Autodesk Fusion 360 part; units mm, degrees
(part 7 of 12)
  line L1818 (4.0736, 136.7487) -> (8.4037, 134.2487)
  line L1819 (8.4037, 134.2487) -> (12.7339, 136.7487)
  line L1820 (12.7339, 136.7487) -> (12.7339, 141.7487)
  line L1821 (12.7339, 141.7487) -> (8.4037, 144.2487)
  line L1822 (19.064, 144.2487) -> (14.7339, 141.7487)
  line L1823 (14.7339, 141.7487) -> (14.7339, 136.7487)
  line L1824 (14.7339, 136.7487) -> (19.064, 134.2487)
  line L1825 (19.064, 134.2487) -> (23.3941, 136.7487)
  line L1826 (23.3941, 136.7487) -> (23.3941, 141.7487)
  line L1827 (23.3941, 141.7487) -> (19.064, 144.2487)
  line L1828 (29.7242, 144.2487) -> (25.3941, 141.7487)
  line L1829 (25.3941, 141.7487) -> (25.3941, 136.7487)
  line L1830 (25.3941, 136.7487) -> (29.7242, 134.2487)
  line L1831 (29.7242, 134.2487) -> (34.0544, 136.7487)
  line L1832 (34.0544, 136.7487) -> (34.0544, 141.7487)
  line L1833 (34.0544, 141.7487) -> (29.7242, 144.2487)
  line L1834 (40.3845, 144.2487) -> (36.0544, 141.7487)
  line L1835 (36.0544, 141.7487) -> (36.0544, 136.7487)
  line L1836 (36.0544, 136.7487) -> (40.3845, 134.2487)
  line L1837 (40.3845, 134.2487) -> (44.7146, 136.7487)
  line L1838 (44.7146, 136.7487) -> (44.7146, 141.7487)
  line L1839 (44.7146, 141.7487) -> (40.3845, 144.2487)
  line L1840 (51.0447, 144.2487) -> (46.7146, 141.7487)
  line L1841 (46.7146, 141.7487) -> (46.7146, 136.7487)
  line L1842 (46.7146, 136.7487) -> (51.0447, 134.2487)
  line L1843 (51.0447, 134.2487) -> (55.3749, 136.7487)
  line L1844 (55.3749, 136.7487) -> (55.3749, 141.7487)
  line L1845 (55.3749, 141.7487) -> (51.0447, 144.2487)
  line L1846 (61.705, 144.2487) -> (57.3749, 141.7487)
  line L1847 (57.3749, 141.7487) -> (57.3749, 136.7487)
  line L1848 (57.3749, 136.7487) -> (61.705, 134.2487)
  line L1849 (61.705, 134.2487) -> (66.0351, 136.7487)
  line L1850 (66.0351, 136.7487) -> (66.0351, 141.7487)
  line L1851 (66.0351, 141.7487) -> (61.705, 144.2487)
  line L1852 (-146.17, 153.4808) -> (-150.5001, 150.9808)
  line L1853 (-150.5001, 150.9808) -> (-150.5001, 145.9808)
  line L1854 (-150.5001, 145.9808) -> (-146.17, 143.4808)
  line L1855 (-146.17, 143.4808) -> (-141.8398, 145.9808)
  line L1856 (-141.8398, 145.9808) -> (-141.8398, 150.9808)
  line L1857 (-141.8398, 150.9808) -> (-146.17, 153.4808)
  line L1858 (-135.5097, 153.4808) -> (-139.8398, 150.9808)
  line L1859 (-139.8398, 150.9808) -> (-139.8398, 145.9808)
  line L1860 (-139.8398, 145.9808) -> (-135.5097, 143.4808)
  line L1861 (-135.5097, 143.4808) -> (-131.1796, 145.9808)
  line L1862 (-131.1796, 145.9808) -> (-131.1796, 150.9808)
  line L1863 (-131.1796, 150.9808) -> (-135.5097, 153.4808)
  line L1864 (-124.8494, 153.4808) -> (-129.1796, 150.9808)
  line L1865 (-129.1796, 150.9808) -> (-129.1796, 145.9808)
  line L1866 (-129.1796, 145.9808) -> (-124.8494, 143.4808)
  line L1867 (-124.8494, 143.4808) -> (-120.5193, 145.9808)
  line L1868 (-120.5193, 145.9808) -> (-120.5193, 150.9808)
  line L1869 (-120.5193, 150.9808) -> (-124.8494, 153.4808)
  line L1870 (-114.1892, 153.4808) -> (-118.5193, 150.9808)
  line L1871 (-118.5193, 150.9808) -> (-118.5193, 145.9808)
  line L1872 (-118.5193, 145.9808) -> (-114.1892, 143.4808)
  line L1873 (-114.1892, 143.4808) -> (-109.8591, 145.9808)
  line L1874 (-109.8591, 145.9808) -> (-109.8591, 150.9808)
  line L1875 (-109.8591, 150.9808) -> (-114.1892, 153.4808)
  line L1876 (-103.5289, 153.4808) -> (-107.8591, 150.9808)
  line L1877 (-107.8591, 150.9808) -> (-107.8591, 145.9808)
  line L1878 (-107.8591, 145.9808) -> (-103.5289, 143.4808)
  line L1879 (-103.5289, 143.4808) -> (-99.1988, 145.9808)
  line L1880 (-99.1988, 145.9808) -> (-99.1988, 150.9808)
  line L1881 (-99.1988, 150.9808) -> (-103.5289, 153.4808)
  line L1882 (-92.8687, 153.4808) -> (-97.1988, 150.9808)
  line L1883 (-97.1988, 150.9808) -> (-97.1988, 145.9808)
  line L1884 (-97.1988, 145.9808) -> (-92.8687, 143.4808)
  line L1885 (-92.8687, 143.4808) -> (-88.5386, 145.9808)
  line L1886 (-88.5386, 145.9808) -> (-88.5386, 150.9808)
  line L1887 (-88.5386, 150.9808) -> (-92.8687, 153.4808)
  line L1888 (-82.2084, 153.4808) -> (-86.5386, 150.9808)
  line L1889 (-86.5386, 150.9808) -> (-86.5386, 145.9808)
  line L1890 (-86.5386, 145.9808) -> (-82.2084, 143.4808)
  line L1891 (-82.2084, 143.4808) -> (-77.8783, 145.9808)
  line L1892 (-77.8783, 145.9808) -> (-77.8783, 150.9808)
  line L1893 (-77.8783, 150.9808) -> (-82.2084, 153.4808)
  line L1894 (-71.5482, 153.4808) -> (-75.8783, 150.9808)
  line L1895 (-75.8783, 150.9808) -> (-75.8783, 145.9808)
  line L1896 (-75.8783, 145.9808) -> (-71.5482, 143.4808)
  line L1897 (-71.5482, 143.4808) -> (-67.218, 145.9808)
  line L1898 (-67.218, 145.9808) -> (-67.218, 150.9808)
  line L1899 (-67.218, 150.9808) -> (-71.5482, 153.4808)
  line L1900 (-60.8879, 153.4808) -> (-65.218, 150.9808)
  line L1901 (-65.218, 150.9808) -> (-65.218, 145.9808)
  line L1902 (-65.218, 145.9808) -> (-60.8879, 143.4808)
  line L1903 (-60.8879, 143.4808) -> (-56.5578, 145.9808)
  line L1904 (-56.5578, 145.9808) -> (-56.5578, 150.9808)
  line L1905 (-56.5578, 150.9808) -> (-60.8879, 153.4808)
  line L1906 (-50.2277, 153.4808) -> (-54.5578, 150.9808)
  line L1907 (-54.5578, 150.9808) -> (-54.5578, 145.9808)
  line L1908 (-54.5578, 145.9808) -> (-50.2277, 143.4808)
  line L1909 (-50.2277, 143.4808) -> (-45.8975, 145.9808)
  line L1910 (-45.8975, 145.9808) -> (-45.8975, 150.9808)
  line L1911 (-45.8975, 150.9808) -> (-50.2277, 153.4808)
  line L1912 (-39.5674, 153.4808) -> (-43.8975, 150.9808)
  line L1913 (-43.8975, 150.9808) -> (-43.8975, 145.9808)
  line L1914 (-43.8975, 145.9808) -> (-39.5674, 143.4808)
  line L1915 (-39.5674, 143.4808) -> (-35.2373, 145.9808)
  line L1916 (-35.2373, 145.9808) -> (-35.2373, 150.9808)
  line L1917 (-35.2373, 150.9808) -> (-39.5674, 153.4808)
  line L1918 (-28.9072, 153.4808) -> (-33.2373, 150.9808)
  line L1919 (-33.2373, 150.9808) -> (-33.2373, 145.9808)
  line L1920 (-33.2373, 145.9808) -> (-28.9072, 143.4808)
  line L1921 (-28.9072, 143.4808) -> (-24.577, 145.9808)
  line L1922 (-24.577, 145.9808) -> (-24.577, 150.9808)
  line L1923 (-24.577, 150.9808) -> (-28.9072, 153.4808)
  line L1924 (-18.2469, 153.4808) -> (-22.577, 150.9808)
  line L1925 (-22.577, 150.9808) -> (-22.577, 145.9808)
  line L1926 (-22.577, 145.9808) -> (-18.2469, 143.4808)
  line L1927 (-18.2469, 143.4808) -> (-13.9168, 145.9808)
  line L1928 (-13.9168, 145.9808) -> (-13.9168, 150.9808)
  line L1929 (-13.9168, 150.9808) -> (-18.2469, 153.4808)
  line L1930 (-7.5866, 153.4808) -> (-11.9168, 150.9808)
  line L1931 (-11.9168, 150.9808) -> (-11.9168, 145.9808)
  line L1932 (-11.9168, 145.9808) -> (-7.5866, 143.4808)
  line L1933 (-7.5866, 143.4808) -> (-3.2565, 145.9808)
  line L1934 (-3.2565, 145.9808) -> (-3.2565, 150.9808)
  line L1935 (-3.2565, 150.9808) -> (-7.5866, 153.4808)
  line L1936 (3.0736, 153.4808) -> (-1.2565, 150.9808)
  line L1937 (-1.2565, 150.9808) -> (-1.2565, 145.9808)
  line L1938 (-1.2565, 145.9808) -> (3.0736, 143.4808)
  line L1939 (3.0736, 143.4808) -> (7.4037, 145.9808)
  line L1940 (7.4037, 145.9808) -> (7.4037, 150.9808)
  line L1941 (7.4037, 150.9808) -> (3.0736, 153.4808)
  line L1942 (13.7339, 153.4808) -> (9.4037, 150.9808)
  line L1943 (9.4037, 150.9808) -> (9.4037, 145.9808)
  line L1944 (9.4037, 145.9808) -> (13.7339, 143.4808)
  line L1945 (13.7339, 143.4808) -> (18.064, 145.9808)
  line L1946 (18.064, 145.9808) -> (18.064, 150.9808)
  line L1947 (18.064, 150.9808) -> (13.7339, 153.4808)
  line L1948 (24.3941, 153.4808) -> (20.064, 150.9808)
  line L1949 (20.064, 150.9808) -> (20.064, 145.9808)
  line L1950 (20.064, 145.9808) -> (24.3941, 143.4808)
  line L1951 (24.3941, 143.4808) -> (28.7242, 145.9808)
  line L1952 (28.7242, 145.9808) -> (28.7242, 150.9808)
  line L1953 (28.7242, 150.9808) -> (24.3941, 153.4808)
  line L1954 (35.0544, 153.4808) -> (30.7242, 150.9808)
  line L1955 (30.7242, 150.9808) -> (30.7242, 145.9808)
  line L1956 (30.7242, 145.9808) -> (35.0544, 143.4808)
  line L1957 (35.0544, 143.4808) -> (39.3845, 145.9808)
  line L1958 (39.3845, 145.9808) -> (39.3845, 150.9808)
  line L1959 (39.3845, 150.9808) -> (35.0544, 153.4808)
  line L1960 (45.7146, 153.4808) -> (41.3845, 150.9808)
  line L1961 (41.3845, 150.9808) -> (41.3845, 145.9808)
  line L1962 (41.3845, 145.9808) -> (45.7146, 143.4808)
  line L1963 (45.7146, 143.4808) -> (50.0447, 145.9808)
  line L1964 (50.0447, 145.9808) -> (50.0447, 150.9808)
  line L1965 (50.0447, 150.9808) -> (45.7146, 153.4808)
  line L1966 (56.3749, 153.4808) -> (52.0447, 150.9808)
  line L1967 (52.0447, 150.9808) -> (52.0447, 145.9808)
  line L1968 (52.0447, 145.9808) -> (56.3749, 143.4808)
  line L1969 (56.3749, 143.4808) -> (60.705, 145.9808)
  line L1970 (60.705, 145.9808) -> (60.705, 150.9808)
  line L1971 (60.705, 150.9808) -> (56.3749, 153.4808)
  line L1972 (-151.5001, 162.7128) -> (-155.8302, 160.2128)
  line L1973 (-155.8302, 160.2128) -> (-155.8302, 155.2128)
  line L1974 (-155.8302, 155.2128) -> (-151.5001, 152.7128)
  line L1975 (-151.5001, 152.7128) -> (-147.17, 155.2128)
  line L1976 (-147.17, 155.2128) -> (-147.17, 160.2128)
  line L1977 (-147.17, 160.2128) -> (-151.5001, 162.7128)
  line L1978 (-140.8398, 162.7128) -> (-145.17, 160.2128)
  line L1979 (-145.17, 160.2128) -> (-145.17, 155.2128)
  line L1980 (-145.17, 155.2128) -> (-140.8398, 152.7128)
  line L1981 (-140.8398, 152.7128) -> (-136.5097, 155.2128)
  line L1982 (-136.5097, 155.2128) -> (-136.5097, 160.2128)
  line L1983 (-136.5097, 160.2128) -> (-140.8398, 162.7128)
  line L1984 (-130.1796, 162.7128) -> (-134.5097, 160.2128)
  line L1985 (-134.5097, 160.2128) -> (-134.5097, 155.2128)
  line L1986 (-134.5097, 155.2128) -> (-130.1796, 152.7128)
  line L1987 (-130.1796, 152.7128) -> (-125.8494, 155.2128)
  line L1988 (-125.8494, 155.2128) -> (-125.8494, 160.2128)
  line L1989 (-125.8494, 160.2128) -> (-130.1796, 162.7128)
  line L1990 (-119.5193, 162.7128) -> (-123.8494, 160.2128)
  line L1991 (-123.8494, 160.2128) -> (-123.8494, 155.2128)
  line L1992 (-123.8494, 155.2128) -> (-119.5193, 152.7128)
  line L1993 (-119.5193, 152.7128) -> (-115.1892, 155.2128)
  line L1994 (-115.1892, 155.2128) -> (-115.1892, 160.2128)
  line L1995 (-115.1892, 160.2128) -> (-119.5193, 162.7128)
  line L1996 (-108.8591, 162.7128) -> (-113.1892, 160.2128)
  line L1997 (-113.1892, 160.2128) -> (-113.1892, 155.2128)
  line L1998 (-113.1892, 155.2128) -> (-108.8591, 152.7128)
  line L1999 (-108.8591, 152.7128) -> (-104.5289, 155.2128)
  line L2000 (-104.5289, 155.2128) -> (-104.5289, 160.2128)
  line L2001 (-104.5289, 160.2128) -> (-108.8591, 162.7128)
  line L2002 (-98.1988, 162.7128) -> (-102.5289, 160.2128)
  line L2003 (-102.5289, 160.2128) -> (-102.5289, 155.2128)
  line L2004 (-102.5289, 155.2128) -> (-98.1988, 152.7128)
  line L2005 (-98.1988, 152.7128) -> (-93.8687, 155.2128)
  line L2006 (-93.8687, 155.2128) -> (-93.8687, 160.2128)
  line L2007 (-93.8687, 160.2128) -> (-98.1988, 162.7128)
  line L2008 (-87.5386, 162.7128) -> (-91.8687, 160.2128)
  line L2009 (-91.8687, 160.2128) -> (-91.8687, 155.2128)
  line L2010 (-91.8687, 155.2128) -> (-87.5386, 152.7128)
  line L2011 (-87.5386, 152.7128) -> (-83.2084, 155.2128)
  line L2012 (-83.2084, 155.2128) -> (-83.2084, 160.2128)
  line L2013 (-83.2084, 160.2128) -> (-87.5386, 162.7128)
  line L2014 (-76.8783, 162.7128) -> (-81.2084, 160.2128)
  line L2015 (-81.2084, 160.2128) -> (-81.2084, 155.2128)
  line L2016 (-81.2084, 155.2128) -> (-76.8783, 152.7128)
  line L2017 (-76.8783, 152.7128) -> (-72.5482, 155.2128)
  line L2018 (-72.5482, 155.2128) -> (-72.5482, 160.2128)
  line L2019 (-72.5482, 160.2128) -> (-76.8783, 162.7128)
  line L2020 (-66.218, 162.7128) -> (-70.5482, 160.2128)
  line L2021 (-70.5482, 160.2128) -> (-70.5482, 155.2128)
  line L2022 (-70.5482, 155.2128) -> (-66.218, 152.7128)
  line L2023 (-66.218, 152.7128) -> (-61.8879, 155.2128)
  line L2024 (-61.8879, 155.2128) -> (-61.8879, 160.2128)
  line L2025 (-61.8879, 160.2128) -> (-66.218, 162.7128)
  line L2026 (-55.5578, 162.7128) -> (-59.8879, 160.2128)
  line L2027 (-59.8879, 160.2128) -> (-59.8879, 155.2128)
  line L2028 (-59.8879, 155.2128) -> (-55.5578, 152.7128)
  line L2029 (-55.5578, 152.7128) -> (-51.2277, 155.2128)
  line L2030 (-51.2277, 155.2128) -> (-51.2277, 160.2128)
  line L2031 (-51.2277, 160.2128) -> (-55.5578, 162.7128)
  line L2032 (-44.8975, 162.7128) -> (-49.2277, 160.2128)
  line L2033 (-49.2277, 160.2128) -> (-49.2277, 155.2128)
  line L2034 (-49.2277, 155.2128) -> (-44.8975, 152.7128)
  line L2035 (-44.8975, 152.7128) -> (-40.5674, 155.2128)
  line L2036 (-40.5674, 155.2128) -> (-40.5674, 160.2128)
  line L2037 (-40.5674, 160.2128) -> (-44.8975, 162.7128)
  line L2038 (-34.2373, 162.7128) -> (-38.5674, 160.2128)
  line L2039 (-38.5674, 160.2128) -> (-38.5674, 155.2128)
  line L2040 (-38.5674, 155.2128) -> (-34.2373, 152.7128)
  line L2041 (-34.2373, 152.7128) -> (-29.9072, 155.2128)
  line L2042 (-29.9072, 155.2128) -> (-29.9072, 160.2128)
  line L2043 (-29.9072, 160.2128) -> (-34.2373, 162.7128)
  line L2044 (-23.577, 162.7128) -> (-27.9072, 160.2128)
  line L2045 (-27.9072, 160.2128) -> (-27.9072, 155.2128)
  line L2046 (-27.9072, 155.2128) -> (-23.577, 152.7128)
  line L2047 (-23.577, 152.7128) -> (-19.2469, 155.2128)
  line L2048 (-19.2469, 155.2128) -> (-19.2469, 160.2128)
  line L2049 (-19.2469, 160.2128) -> (-23.577, 162.7128)
  line L2050 (-12.9168, 162.7128) -> (-17.2469, 160.2128)
  line L2051 (-17.2469, 160.2128) -> (-17.2469, 155.2128)
  line L2052 (-17.2469, 155.2128) -> (-12.9168, 152.7128)
  line L2053 (-12.9168, 152.7128) -> (-8.5866, 155.2128)
  line L2054 (-8.5866, 155.2128) -> (-8.5866, 160.2128)
  line L2055 (-8.5866, 160.2128) -> (-12.9168, 162.7128)
  line L2056 (-2.2565, 162.7128) -> (-6.5866, 160.2128)
  line L2057 (-6.5866, 160.2128) -> (-6.5866, 155.2128)
  line L2058 (-6.5866, 155.2128) -> (-2.2565, 152.7128)
  line L2059 (-2.2565, 152.7128) -> (2.0736, 155.2128)
  line L2060 (2.0736, 155.2128) -> (2.0736, 160.2128)
  line L2061 (2.0736, 160.2128) -> (-2.2565, 162.7128)
  line L2062 (8.4037, 162.7128) -> (4.0736, 160.2128)
  line L2063 (4.0736, 160.2128) -> (4.0736, 155.2128)
  line L2064 (4.0736, 155.2128) -> (8.4037, 152.7128)
  line L2065 (8.4037, 152.7128) -> (12.7339, 155.2128)
  line L2066 (12.7339, 155.2128) -> (12.7339, 160.2128)
  line L2067 (12.7339, 160.2128) -> (8.4037, 162.7128)
  line L2068 (19.064, 162.7128) -> (14.7339, 160.2128)
  line L2069 (14.7339, 160.2128) -> (14.7339, 155.2128)
  line L2070 (14.7339, 155.2128) -> (19.064, 152.7128)
  line L2071 (19.064, 152.7128) -> (23.3941, 155.2128)
  line L2072 (23.3941, 155.2128) -> (23.3941, 160.2128)
  line L2073 (23.3941, 160.2128) -> (19.064, 162.7128)
  line L2074 (29.7242, 162.7128) -> (25.3941, 160.2128)
  line L2075 (25.3941, 160.2128) -> (25.3941, 155.2128)
  line L2076 (25.3941, 155.2128) -> (29.7242, 152.7128)
  line L2077 (29.7242, 152.7128) -> (34.0544, 155.2128)
  line L2078 (34.0544, 155.2128) -> (34.0544, 160.2128)
  line L2079 (34.0544, 160.2128) -> (29.7242, 162.7128)
  line L2080 (40.3845, 162.7128) -> (36.0544, 160.2128)
  line L2081 (36.0544, 160.2128) -> (36.0544, 155.2128)
  line L2082 (36.0544, 155.2128) -> (40.3845, 152.7128)
  line L2083 (40.3845, 152.7128) -> (44.7146, 155.2128)
  line L2084 (44.7146, 155.2128) -> (44.7146, 160.2128)
  line L2085 (44.7146, 160.2128) -> (40.3845, 162.7128)
  line L2086 (51.0447, 162.7128) -> (46.7146, 160.2128)
  line L2087 (46.7146, 160.2128) -> (46.7146, 155.2128)
  line L2088 (46.7146, 155.2128) -> (51.0447, 152.7128)
  line L2089 (51.0447, 152.7128) -> (55.3749, 155.2128)
  line L2090 (55.3749, 155.2128) -> (55.3749, 160.2128)
  line L2091 (55.3749, 160.2128) -> (51.0447, 162.7128)
  line L2092 (61.705, 162.7128) -> (57.3749, 160.2128)
  line L2093 (57.3749, 160.2128) -> (57.3749, 155.2128)
  line L2094 (57.3749, 155.2128) -> (61.705, 152.7128)
  line L2095 (61.705, 152.7128) -> (66.0351, 155.2128)
  line L2096 (66.0351, 155.2128) -> (66.0351, 160.2128)
  line L2097 (66.0351, 160.2128) -> (61.705, 162.7128)
  line L2098 (-146.17, 171.9449) -> (-150.5001, 169.4449)
  line L2099 (-150.5001, 169.4449) -> (-150.5001, 164.4449)
  line L2100 (-150.5001, 164.4449) -> (-146.17, 161.9449)
  line L2101 (-146.17, 161.9449) -> (-141.8398, 164.4449)
  line L2102 (-141.8398, 164.4449) -> (-141.8398, 169.4449)
  line L2103 (-141.8398, 169.4449) -> (-146.17, 171.9449)
  line L2104 (-135.5097, 171.9449) -> (-139.8398, 169.4449)
  line L2105 (-139.8398, 169.4449) -> (-139.8398, 164.4449)
  line L2106 (-139.8398, 164.4449) -> (-135.5097, 161.9449)
  line L2107 (-135.5097, 161.9449) -> (-131.1796, 164.4449)
  line L2108 (-131.1796, 164.4449) -> (-131.1796, 169.4449)
  line L2109 (-131.1796, 169.4449) -> (-135.5097, 171.9449)
  line L2110 (-124.8494, 171.9449) -> (-129.1796, 169.4449)
  line L2111 (-129.1796, 169.4449) -> (-129.1796, 164.4449)
  line L2112 (-129.1796, 164.4449) -> (-124.8494, 161.9449)
  line L2113 (-124.8494, 161.9449) -> (-120.5193, 164.4449)
  line L2114 (-120.5193, 164.4449) -> (-120.5193, 169.4449)
  line L2115 (-120.5193, 169.4449) -> (-124.8494, 171.9449)
  line L2116 (-114.1892, 171.9449) -> (-118.5193, 169.4449)
  line L2117 (-118.5193, 169.4449) -> (-118.5193, 164.4449)
  line L2118 (-118.5193, 164.4449) -> (-114.1892, 161.9449)
  line L2119 (-114.1892, 161.9449) -> (-109.8591, 164.4449)
  line L2120 (-109.8591, 164.4449) -> (-109.8591, 169.4449)
  line L2121 (-109.8591, 169.4449) -> (-114.1892, 171.9449)
  line L2122 (-103.5289, 171.9449) -> (-107.8591, 169.4449)
  line L2123 (-107.8591, 169.4449) -> (-107.8591, 164.4449)
  line L2124 (-107.8591, 164.4449) -> (-103.5289, 161.9449)
  line L2125 (-103.5289, 161.9449) -> (-99.1988, 164.4449)
  line L2126 (-99.1988, 164.4449) -> (-99.1988, 169.4449)
  line L2127 (-99.1988, 169.4449) -> (-103.5289, 171.9449)
  line L2128 (-92.8687, 171.9449) -> (-97.1988, 169.4449)
  line L2129 (-97.1988, 169.4449) -> (-97.1988, 164.4449)
  line L2130 (-97.1988, 164.4449) -> (-92.8687, 161.9449)
  line L2131 (-92.8687, 161.9449) -> (-88.5386, 164.4449)
  line L2132 (-88.5386, 164.4449) -> (-88.5386, 169.4449)
  line L2133 (-88.5386, 169.4449) -> (-92.8687, 171.9449)
  line L2134 (-82.2084, 171.9449) -> (-86.5386, 169.4449)
  line L2135 (-86.5386, 169.4449) -> (-86.5386, 164.4449)
  line L2136 (-86.5386, 164.4449) -> (-82.2084, 161.9449)
  line L2137 (-82.2084, 161.9449) -> (-77.8783, 164.4449)
  line L2138 (-77.8783, 164.4449) -> (-77.8783, 169.4449)
  line L2139 (-77.8783, 169.4449) -> (-82.2084, 171.9449)
  line L2140 (-71.5482, 171.9449) -> (-75.8783, 169.4449)
  line L2141 (-75.8783, 169.4449) -> (-75.8783, 164.4449)
  line L2142 (-75.8783, 164.4449) -> (-71.5482, 161.9449)
  line L2143 (-71.5482, 161.9449) -> (-67.218, 164.4449)
  line L2144 (-67.218, 164.4449) -> (-67.218, 169.4449)
  line L2145 (-67.218, 169.4449) -> (-71.5482, 171.9449)
  line L2146 (-60.8879, 171.9449) -> (-65.218, 169.4449)
  line L2147 (-65.218, 169.4449) -> (-65.218, 164.4449)
  line L2148 (-65.218, 164.4449) -> (-60.8879, 161.9449)
  line L2149 (-60.8879, 161.9449) -> (-56.5578, 164.4449)
  line L2150 (-56.5578, 164.4449) -> (-56.5578, 169.4449)
  line L2151 (-56.5578, 169.4449) -> (-60.8879, 171.9449)
  line L2152 (-50.2277, 171.9449) -> (-54.5578, 169.4449)
  line L2153 (-54.5578, 169.4449) -> (-54.5578, 164.4449)
  line L2154 (-54.5578, 164.4449) -> (-50.2277, 161.9449)
  line L2155 (-50.2277, 161.9449) -> (-45.8975, 164.4449)
  line L2156 (-45.8975, 164.4449) -> (-45.8975, 169.4449)
  line L2157 (-45.8975, 169.4449) -> (-50.2277, 171.9449)
  line L2158 (-39.5674, 171.9449) -> (-43.8975, 169.4449)
  line L2159 (-43.8975, 169.4449) -> (-43.8975, 164.4449)
  line L2160 (-43.8975, 164.4449) -> (-39.5674, 161.9449)
  line L2161 (-39.5674, 161.9449) -> (-35.2373, 164.4449)
  line L2162 (-35.2373, 164.4449) -> (-35.2373, 169.4449)
  line L2163 (-35.2373, 169.4449) -> (-39.5674, 171.9449)
  line L2164 (-28.9072, 171.9449) -> (-33.2373, 169.4449)
  line L2165 (-33.2373, 169.4449) -> (-33.2373, 164.4449)
  line L2166 (-33.2373, 164.4449) -> (-28.9072, 161.9449)
  line L2167 (-28.9072, 161.9449) -> (-24.577, 164.4449)
  line L2168 (-24.577, 164.4449) -> (-24.577, 169.4449)
  line L2169 (-24.577, 169.4449) -> (-28.9072, 171.9449)
  line L2170 (-18.2469, 171.9449) -> (-22.577, 169.4449)
  line L2171 (-22.577, 169.4449) -> (-22.577, 164.4449)
  line L2172 (-22.577, 164.4449) -> (-18.2469, 161.9449)
  line L2173 (-18.2469, 161.9449) -> (-13.9168, 164.4449)
  line L2174 (-13.9168, 164.4449) -> (-13.9168, 169.4449)
  line L2175 (-13.9168, 169.4449) -> (-18.2469, 171.9449)
  line L2176 (-7.5866, 171.9449) -> (-11.9168, 169.4449)
  line L2177 (-11.9168, 169.4449) -> (-11.9168, 164.4449)
  line L2178 (-11.9168, 164.4449) -> (-7.5866, 161.9449)
  line L2179 (-7.5866, 161.9449) -> (-3.2565, 164.4449)
  line L2180 (-3.2565, 164.4449) -> (-3.2565, 169.4449)
  line L2181 (-3.2565, 169.4449) -> (-7.5866, 171.9449)
  line L2182 (3.0736, 171.9449) -> (-1.2565, 169.4449)
  line L2183 (-1.2565, 169.4449) -> (-1.2565, 164.4449)
  line L2184 (-1.2565, 164.4449) -> (3.0736, 161.9449)
  line L2185 (3.0736, 161.9449) -> (7.4037, 164.4449)
  line L2186 (7.4037, 164.4449) -> (7.4037, 169.4449)
  line L2187 (7.4037, 169.4449) -> (3.0736, 171.9449)
  line L2188 (13.7339, 171.9449) -> (9.4037, 169.4449)
  line L2189 (9.4037, 169.4449) -> (9.4037, 164.4449)
  line L2190 (9.4037, 164.4449) -> (13.7339, 161.9449)
  line L2191 (13.7339, 161.9449) -> (18.064, 164.4449)
  line L2192 (18.064, 164.4449) -> (18.064, 169.4449)
  line L2193 (18.064, 169.4449) -> (13.7339, 171.9449)
  line L2194 (24.3941, 171.9449) -> (20.064, 169.4449)
  line L2195 (20.064, 169.4449) -> (20.064, 164.4449)
  line L2196 (20.064, 164.4449) -> (24.3941, 161.9449)
  line L2197 (24.3941, 161.9449) -> (28.7242, 164.4449)
  line L2198 (28.7242, 164.4449) -> (28.7242, 169.4449)
  line L2199 (28.7242, 169.4449) -> (24.3941, 171.9449)
  line L2200 (35.0544, 171.9449) -> (30.7242, 169.4449)
  line L2201 (30.7242, 169.4449) -> (30.7242, 164.4449)
  line L2202 (30.7242, 164.4449) -> (35.0544, 161.9449)
  line L2203 (35.0544, 161.9449) -> (39.3845, 164.4449)
  line L2204 (39.3845, 164.4449) -> (39.3845, 169.4449)
  line L2205 (39.3845, 169.4449) -> (35.0544, 171.9449)
  line L2206 (45.7146, 171.9449) -> (41.3845, 169.4449)
  line L2207 (41.3845, 169.4449) -> (41.3845, 164.4449)
  line L2208 (41.3845, 164.4449) -> (45.7146, 161.9449)
  line L2209 (45.7146, 161.9449) -> (50.0447, 164.4449)
  line L2210 (50.0447, 164.4449) -> (50.0447, 169.4449)
  line L2211 (50.0447, 169.4449) -> (45.7146, 171.9449)
  line L2212 (56.3749, 171.9449) -> (52.0447, 169.4449)
  line L2213 (52.0447, 169.4449) -> (52.0447, 164.4449)
  line L2214 (52.0447, 164.4449) -> (56.3749, 161.9449)
  line L2215 (56.3749, 161.9449) -> (60.705, 164.4449)
  line L2216 (60.705, 164.4449) -> (60.705, 169.4449)
  line L2217 (60.705, 169.4449) -> (56.3749, 171.9449)
  line L2218 (-151.5001, 181.1769) -> (-155.8302, 178.6769)
  line L2219 (-155.8302, 178.6769) -> (-155.8302, 173.6769)
  line L2220 (-155.8302, 173.6769) -> (-151.5001, 171.1769)
  line L2221 (-151.5001, 171.1769) -> (-147.17, 173.6769)
  line L2222 (-147.17, 173.6769) -> (-147.17, 178.6769)
  line L2223 (-147.17, 178.6769) -> (-151.5001, 181.1769)
  line L2224 (-140.8398, 181.1769) -> (-145.17, 178.6769)
  line L2225 (-145.17, 178.6769) -> (-145.17, 173.6769)
  line L2226 (-145.17, 173.6769) -> (-140.8398, 171.1769)
  line L2227 (-140.8398, 171.1769) -> (-136.5097, 173.6769)
  line L2228 (-136.5097, 173.6769) -> (-136.5097, 178.6769)
  line L2229 (-136.5097, 178.6769) -> (-140.8398, 181.1769)
  line L2230 (-130.1796, 181.1769) -> (-134.5097, 178.6769)
  line L2231 (-134.5097, 178.6769) -> (-134.5097, 173.6769)
  line L2232 (-134.5097, 173.6769) -> (-130.1796, 171.1769)
  line L2233 (-130.1796, 171.1769) -> (-125.8494, 173.6769)
  line L2234 (-125.8494, 173.6769) -> (-125.8494, 178.6769)
  line L2235 (-125.8494, 178.6769) -> (-130.1796, 181.1769)
  line L2236 (-119.5193, 181.1769) -> (-123.8494, 178.6769)
  line L2237 (-123.8494, 178.6769) -> (-123.8494, 173.6769)
  line L2238 (-123.8494, 173.6769) -> (-119.5193, 171.1769)
  line L2239 (-119.5193, 171.1769) -> (-115.1892, 173.6769)
  line L2240 (-115.1892, 173.6769) -> (-115.1892, 178.6769)
  line L2241 (-115.1892, 178.6769) -> (-119.5193, 181.1769)
  line L2242 (-108.8591, 181.1769) -> (-113.1892, 178.6769)
  line L2243 (-113.1892, 178.6769) -> (-113.1892, 173.6769)
  line L2244 (-113.1892, 173.6769) -> (-108.8591, 171.1769)
  line L2245 (-108.8591, 171.1769) -> (-104.5289, 173.6769)
  line L2246 (-104.5289, 173.6769) -> (-104.5289, 178.6769)
  line L2247 (-104.5289, 178.6769) -> (-108.8591, 181.1769)
  line L2248 (-98.1988, 181.1769) -> (-102.5289, 178.6769)
  line L2249 (-102.5289, 178.6769) -> (-102.5289, 173.6769)
  line L2250 (-102.5289, 173.6769) -> (-98.1988, 171.1769)
  line L2251 (-98.1988, 171.1769) -> (-93.8687, 173.6769)
  line L2252 (-93.8687, 173.6769) -> (-93.8687, 178.6769)
  line L2253 (-93.8687, 178.6769) -> (-98.1988, 181.1769)
  line L2254 (-87.5386, 181.1769) -> (-91.8687, 178.6769)
  line L2255 (-91.8687, 178.6769) -> (-91.8687, 173.6769)
  line L2256 (-91.8687, 173.6769) -> (-87.5386, 171.1769)
  line L2257 (-87.5386, 171.1769) -> (-83.2084, 173.6769)
  line L2258 (-83.2084, 173.6769) -> (-83.2084, 178.6769)
  line L2259 (-83.2084, 178.6769) -> (-87.5386, 181.1769)
  line L2260 (-76.8783, 181.1769) -> (-81.2084, 178.6769)
  line L2261 (-81.2084, 178.6769) -> (-81.2084, 173.6769)
  line L2262 (-81.2084, 173.6769) -> (-76.8783, 171.1769)
  line L2263 (-76.8783, 171.1769) -> (-72.5482, 173.6769)
  line L2264 (-72.5482, 173.6769) -> (-72.5482, 178.6769)
  line L2265 (-72.5482, 178.6769) -> (-76.8783, 181.1769)
  line L2266 (-66.218, 181.1769) -> (-70.5482, 178.6769)
  line L2267 (-70.5482, 178.6769) -> (-70.5482, 173.6769)
  line L2268 (-70.5482, 173.6769) -> (-66.218, 171.1769)
  line L2269 (-66.218, 171.1769) -> (-61.8879, 173.6769)
  line L2270 (-61.8879, 173.6769) -> (-61.8879, 178.6769)
  line L2271 (-61.8879, 178.6769) -> (-66.218, 181.1769)
  line L2272 (-55.5578, 181.1769) -> (-59.8879, 178.6769)
  line L2273 (-59.8879, 178.6769) -> (-59.8879, 173.6769)
  line L2274 (-59.8879, 173.6769) -> (-55.5578, 171.1769)
  line L2275 (-55.5578, 171.1769) -> (-51.2277, 173.6769)
  line L2276 (-51.2277, 173.6769) -> (-51.2277, 178.6769)
  line L2277 (-51.2277, 178.6769) -> (-55.5578, 181.1769)
  line L2278 (-44.8975, 181.1769) -> (-49.2277, 178.6769)
  line L2279 (-49.2277, 178.6769) -> (-49.2277, 173.6769)
  line L2280 (-49.2277, 173.6769) -> (-44.8975, 171.1769)
  line L2281 (-44.8975, 171.1769) -> (-40.5674, 173.6769)
  line L2282 (-40.5674, 173.6769) -> (-40.5674, 178.6769)
  line L2283 (-40.5674, 178.6769) -> (-44.8975, 181.1769)
  line L2284 (-34.2373, 181.1769) -> (-38.5674, 178.6769)
  line L2285 (-38.5674, 178.6769) -> (-38.5674, 173.6769)
  line L2286 (-38.5674, 173.6769) -> (-34.2373, 171.1769)
  line L2287 (-34.2373, 171.1769) -> (-29.9072, 173.6769)
  line L2288 (-29.9072, 173.6769) -> (-29.9072, 178.6769)
  line L2289 (-29.9072, 178.6769) -> (-34.2373, 181.1769)
  line L2290 (-23.577, 181.1769) -> (-27.9072, 178.6769)
  line L2291 (-27.9072, 178.6769) -> (-27.9072, 173.6769)
  line L2292 (-27.9072, 173.6769) -> (-23.577, 171.1769)
  line L2293 (-23.577, 171.1769) -> (-19.2469, 173.6769)
  line L2294 (-19.2469, 173.6769) -> (-19.2469, 178.6769)
  line L2295 (-19.2469, 178.6769) -> (-23.577, 181.1769)
  line L2296 (-12.9168, 181.1769) -> (-17.2469, 178.6769)
  line L2297 (-17.2469, 178.6769) -> (-17.2469, 173.6769)
  line L2298 (-17.2469, 173.6769) -> (-12.9168, 171.1769)
  line L2299 (-12.9168, 171.1769) -> (-8.5866, 173.6769)
  line L2300 (-8.5866, 173.6769) -> (-8.5866, 178.6769)
  line L2301 (-8.5866, 178.6769) -> (-12.9168, 181.1769)
  line L2302 (-2.2565, 181.1769) -> (-6.5866, 178.6769)
  line L2303 (-6.5866, 178.6769) -> (-6.5866, 173.6769)
  line L2304 (-6.5866, 173.6769) -> (-2.2565, 171.1769)
  line L2305 (-2.2565, 171.1769) -> (2.0736, 173.6769)
  line L2306 (2.0736, 173.6769) -> (2.0736, 178.6769)
  line L2307 (2.0736, 178.6769) -> (-2.2565, 181.1769)
  line L2308 (8.4037, 181.1769) -> (4.0736, 178.6769)
  line L2309 (4.0736, 178.6769) -> (4.0736, 173.6769)
  line L2310 (4.0736, 173.6769) -> (8.4037, 171.1769)
  line L2311 (8.4037, 171.1769) -> (12.7339, 173.6769)
  line L2312 (12.7339, 173.6769) -> (12.7339, 178.6769)
  line L2313 (12.7339, 178.6769) -> (8.4037, 181.1769)
  line L2314 (19.064, 181.1769) -> (14.7339, 178.6769)
  line L2315 (14.7339, 178.6769) -> (14.7339, 173.6769)
  line L2316 (14.7339, 173.6769) -> (19.064, 171.1769)
  line L2317 (19.064, 171.1769) -> (23.3941, 173.6769)
  line L2318 (23.3941, 173.6769) -> (23.3941, 178.6769)
  line L2319 (23.3941, 178.6769) -> (19.064, 181.1769)
  line L2320 (29.7242, 181.1769) -> (25.3941, 178.6769)
  line L2321 (25.3941, 178.6769) -> (25.3941, 173.6769)
  line L2322 (25.3941, 173.6769) -> (29.7242, 171.1769)
  line L2323 (29.7242, 171.1769) -> (34.0544, 173.6769)
  line L2324 (34.0544, 173.6769) -> (34.0544, 178.6769)
  line L2325 (34.0544, 178.6769) -> (29.7242, 181.1769)
  line L2326 (40.3845, 181.1769) -> (36.0544, 178.6769)
  line L2327 (36.0544, 178.6769) -> (36.0544, 173.6769)
  line L2328 (36.0544, 173.6769) -> (40.3845, 171.1769)
  line L2329 (40.3845, 171.1769) -> (44.7146, 173.6769)
  line L2330 (44.7146, 173.6769) -> (44.7146, 178.6769)
  line L2331 (44.7146, 178.6769) -> (40.3845, 181.1769)
  line L2332 (51.0447, 181.1769) -> (46.7146, 178.6769)
  line L2333 (46.7146, 178.6769) -> (46.7146, 173.6769)
  line L2334 (46.7146, 173.6769) -> (51.0447, 171.1769)
  line L2335 (51.0447, 171.1769) -> (55.3749, 173.6769)
  line L2336 (55.3749, 173.6769) -> (55.3749, 178.6769)
  line L2337 (55.3749, 178.6769) -> (51.0447, 181.1769)
  line L2338 (61.705, 181.1769) -> (57.3749, 178.6769)
  line L2339 (57.3749, 178.6769) -> (57.3749, 173.6769)
  line L2340 (57.3749, 173.6769) -> (61.705, 171.1769)
  line L2341 (61.705, 171.1769) -> (66.0351, 173.6769)
  line L2342 (66.0351, 173.6769) -> (66.0351, 178.6769)
  line L2343 (66.0351, 178.6769) -> (61.705, 181.1769)
  line L2344 (-146.17, 190.409) -> (-150.5001, 187.909)
  line L2345 (-150.5001, 187.909) -> (-150.5001, 182.909)
  line L2346 (-150.5001, 182.909) -> (-146.17, 180.409)
  line L2347 (-146.17, 180.409) -> (-141.8398, 182.909)
  line L2348 (-141.8398, 182.909) -> (-141.8398, 187.909)
  line L2349 (-141.8398, 187.909) -> (-146.17, 190.409)
  line L2350 (-135.5097, 190.409) -> (-139.8398, 187.909)
  line L2351 (-139.8398, 187.909) -> (-139.8398, 182.909)
  line L2352 (-139.8398, 182.909) -> (-135.5097, 180.409)
  line L2353 (-135.5097, 180.409) -> (-131.1796, 182.909)
  line L2354 (-131.1796, 182.909) -> (-131.1796, 187.909)
  line L2355 (-131.1796, 187.909) -> (-135.5097, 190.409)
  line L2356 (-124.8494, 190.409) -> (-129.1796, 187.909)
  line L2357 (-129.1796, 187.909) -> (-129.1796, 182.909)
  line L2358 (-129.1796, 182.909) -> (-124.8494, 180.409)
  line L2359 (-124.8494, 180.409) -> (-120.5193, 182.909)
  line L2360 (-120.5193, 182.909) -> (-120.5193, 187.909)
  line L2361 (-120.5193, 187.909) -> (-124.8494, 190.409)
  line L2362 (-114.1892, 190.409) -> (-118.5193, 187.909)
  line L2363 (-118.5193, 187.909) -> (-118.5193, 182.909)
  line L2364 (-118.5193, 182.909) -> (-114.1892, 180.409)
  line L2365 (-114.1892, 180.409) -> (-109.8591, 182.909)
  line L2366 (-109.8591, 182.909) -> (-109.8591, 187.909)
  line L2367 (-109.8591, 187.909) -> (-114.1892, 190.409)
  line L2368 (-103.5289, 190.409) -> (-107.8591, 187.909)
  line L2369 (-107.8591, 187.909) -> (-107.8591, 182.909)
  line L2370 (-107.8591, 182.909) -> (-103.5289, 180.409)
  line L2371 (-103.5289, 180.409) -> (-99.1988, 182.909)
  line L2372 (-99.1988, 182.909) -> (-99.1988, 187.909)
  line L2373 (-99.1988, 187.909) -> (-103.5289, 190.409)
  line L2374 (-92.8687, 190.409) -> (-97.1988, 187.909)
  line L2375 (-97.1988, 187.909) -> (-97.1988, 182.909)
  line L2376 (-97.1988, 182.909) -> (-92.8687, 180.409)
  line L2377 (-92.8687, 180.409) -> (-88.5386, 182.909)
  line L2378 (-88.5386, 182.909) -> (-88.5386, 187.909)
  line L2379 (-88.5386, 187.909) -> (-92.8687, 190.409)
  line L2380 (-82.2084, 190.409) -> (-86.5386, 187.909)
  line L2381 (-86.5386, 187.909) -> (-86.5386, 182.909)
  line L2382 (-86.5386, 182.909) -> (-82.2084, 180.409)
  line L2383 (-82.2084, 180.409) -> (-77.8783, 182.909)
  line L2384 (-77.8783, 182.909) -> (-77.8783, 187.909)
  line L2385 (-77.8783, 187.909) -> (-82.2084, 190.409)
  line L2386 (-71.5482, 190.409) -> (-75.8783, 187.909)
  line L2387 (-75.8783, 187.909) -> (-75.8783, 182.909)
  line L2388 (-75.8783, 182.909) -> (-71.5482, 180.409)
  line L2389 (-71.5482, 180.409) -> (-67.218, 182.909)
  line L2390 (-67.218, 182.909) -> (-67.218, 187.909)
  line L2391 (-67.218, 187.909) -> (-71.5482, 190.409)
  line L2392 (-60.8879, 190.409) -> (-65.218, 187.909)
  line L2393 (-65.218, 187.909) -> (-65.218, 182.909)
  line L2394 (-65.218, 182.909) -> (-60.8879, 180.409)
  line L2395 (-60.8879, 180.409) -> (-56.5578, 182.909)
  line L2396 (-56.5578, 182.909) -> (-56.5578, 187.909)
  line L2397 (-56.5578, 187.909) -> (-60.8879, 190.409)
  line L2398 (-50.2277, 190.409) -> (-54.5578, 187.909)
  line L2399 (-54.5578, 187.909) -> (-54.5578, 182.909)
  line L2400 (-54.5578, 182.909) -> (-50.2277, 180.409)
  line L2401 (-50.2277, 180.409) -> (-45.8975, 182.909)
  line L2402 (-45.8975, 182.909) -> (-45.8975, 187.909)
  line L2403 (-45.8975, 187.909) -> (-50.2277, 190.409)
  line L2404 (-39.5674, 190.409) -> (-43.8975, 187.909)
  line L2405 (-43.8975, 187.909) -> (-43.8975, 182.909)
  line L2406 (-43.8975, 182.909) -> (-39.5674, 180.409)
  line L2407 (-39.5674, 180.409) -> (-35.2373, 182.909)
  line L2408 (-35.2373, 182.909) -> (-35.2373, 187.909)
  line L2409 (-35.2373, 187.909) -> (-39.5674, 190.409)
  line L2410 (-28.9072, 190.409) -> (-33.2373, 187.909)
  line L2411 (-33.2373, 187.909) -> (-33.2373, 182.909)
  line L2412 (-33.2373, 182.909) -> (-28.9072, 180.409)
  line L2413 (-28.9072, 180.409) -> (-24.577, 182.909)
  line L2414 (-24.577, 182.909) -> (-24.577, 187.909)
  line L2415 (-24.577, 187.909) -> (-28.9072, 190.409)
  line L2416 (-18.2469, 190.409) -> (-22.577, 187.909)
  line L2417 (-22.577, 187.909) -> (-22.577, 182.909)
  line L2418 (-22.577, 182.909) -> (-18.2469, 180.409)
  line L2419 (-18.2469, 180.409) -> (-13.9168, 182.909)
  line L2420 (-13.9168, 182.909) -> (-13.9168, 187.909)
  line L2421 (-13.9168, 187.909) -> (-18.2469, 190.409)
  line L2422 (-7.5866, 190.409) -> (-11.9168, 187.909)
  line L2423 (-11.9168, 187.909) -> (-11.9168, 182.909)
  line L2424 (-11.9168, 182.909) -> (-7.5866, 180.409)
  line L2425 (-7.5866, 180.409) -> (-3.2565, 182.909)
  line L2426 (-3.2565, 182.909) -> (-3.2565, 187.909)
  line L2427 (-3.2565, 187.909) -> (-7.5866, 190.409)
  line L2428 (3.0736, 190.409) -> (-1.2565, 187.909)
  line L2429 (-1.2565, 187.909) -> (-1.2565, 182.909)
  line L2430 (-1.2565, 182.909) -> (3.0736, 180.409)
  line L2431 (3.0736, 180.409) -> (7.4037, 182.909)
  line L2432 (7.4037, 182.909) -> (7.4037, 187.909)
  line L2433 (7.4037, 187.909) -> (3.0736, 190.409)
  line L2434 (13.7339, 190.409) -> (9.4037, 187.909)
  line L2435 (9.4037, 187.909) -> (9.4037, 182.909)
  line L2436 (9.4037, 182.909) -> (13.7339, 180.409)
  line L2437 (13.7339, 180.409) -> (18.064, 182.909)
  line L2438 (18.064, 182.909) -> (18.064, 187.909)
  line L2439 (18.064, 187.909) -> (13.7339, 190.409)
  line L2440 (24.3941, 190.409) -> (20.064, 187.909)
  line L2441 (20.064, 187.909) -> (20.064, 182.909)
  line L2442 (20.064, 182.909) -> (24.3941, 180.409)
  line L2443 (24.3941, 180.409) -> (28.7242, 182.909)
  line L2444 (28.7242, 182.909) -> (28.7242, 187.909)
  line L2445 (28.7242, 187.909) -> (24.3941, 190.409)
  line L2446 (35.0544, 190.409) -> (30.7242, 187.909)
  line L2447 (30.7242, 187.909) -> (30.7242, 182.909)
  line L2448 (30.7242, 182.909) -> (35.0544, 180.409)
  line L2449 (35.0544, 180.409) -> (39.3845, 182.909)
  line L2450 (39.3845, 182.909) -> (39.3845, 187.909)
  line L2451 (39.3845, 187.909) -> (35.0544, 190.409)
  line L2452 (45.7146, 190.409) -> (41.3845, 187.909)
  line L2453 (41.3845, 187.909) -> (41.3845, 182.909)
  line L2454 (41.3845, 182.909) -> (45.7146, 180.409)
  line L2455 (45.7146, 180.409) -> (50.0447, 182.909)
  line L2456 (50.0447, 182.909) -> (50.0447, 187.909)
  line L2457 (50.0447, 187.909) -> (45.7146, 190.409)
  line L2458 (56.3749, 190.409) -> (52.0447, 187.909)
  line L2459 (52.0447, 187.909) -> (52.0447, 182.909)
  line L2460 (52.0447, 182.909) -> (56.3749, 180.409)
  line L2461 (56.3749, 180.409) -> (60.705, 182.909)
  line L2462 (60.705, 182.909) -> (60.705, 187.909)
  line L2463 (60.705, 187.909) -> (56.3749, 190.409)
  line L2464 (-151.5001, 199.641) -> (-155.8302, 197.141)
  line L2465 (-155.8302, 197.141) -> (-155.8302, 192.141)
  line L2466 (-155.8302, 192.141) -> (-151.5001, 189.641)
  line L2467 (-151.5001, 189.641) -> (-147.17, 192.141)
  line L2468 (-147.17, 192.141) -> (-147.17, 197.141)
  line L2469 (-147.17, 197.141) -> (-151.5001, 199.641)
  line L2470 (-140.8398, 199.641) -> (-145.17, 197.141)
  line L2471 (-145.17, 197.141) -> (-145.17, 192.141)
  line L2472 (-145.17, 192.141) -> (-140.8398, 189.641)
  line L2473 (-140.8398, 189.641) -> (-136.5097, 192.141)
  line L2474 (-136.5097, 192.141) -> (-136.5097, 197.141)
  line L2475 (-136.5097, 197.141) -> (-140.8398, 199.641)
  line L2476 (-130.1796, 199.641) -> (-134.5097, 197.141)
  line L2477 (-134.5097, 197.141) -> (-134.5097, 192.141)
  line L2478 (-134.5097, 192.141) -> (-130.1796, 189.641)
  line L2479 (-130.1796, 189.641) -> (-125.8494, 192.141)
  line L2480 (-125.8494, 192.141) -> (-125.8494, 197.141)
  line L2481 (-125.8494, 197.141) -> (-130.1796, 199.641)
  line L2482 (-119.5193, 199.641) -> (-123.8494, 197.141)
  line L2483 (-123.8494, 197.141) -> (-123.8494, 192.141)
  line L2484 (-123.8494, 192.141) -> (-119.5193, 189.641)
  line L2485 (-119.5193, 189.641) -> (-115.1892, 192.141)
  line L2486 (-115.1892, 192.141) -> (-115.1892, 197.141)
  line L2487 (-115.1892, 197.141) -> (-119.5193, 199.641)
  line L2488 (-108.8591, 199.641) -> (-113.1892, 197.141)
  line L2489 (-113.1892, 197.141) -> (-113.1892, 192.141)
  line L2490 (-113.1892, 192.141) -> (-108.8591, 189.641)
  line L2491 (-108.8591, 189.641) -> (-104.5289, 192.141)
  line L2492 (-104.5289, 192.141) -> (-104.5289, 197.141)
  line L2493 (-104.5289, 197.141) -> (-108.8591, 199.641)
  line L2494 (-98.1988, 199.641) -> (-102.5289, 197.141)
  line L2495 (-102.5289, 197.141) -> (-102.5289, 192.141)
  line L2496 (-102.5289, 192.141) -> (-98.1988, 189.641)
  line L2497 (-98.1988, 189.641) -> (-93.8687, 192.141)
  line L2498 (-93.8687, 192.141) -> (-93.8687, 197.141)
  line L2499 (-93.8687, 197.141) -> (-98.1988, 199.641)
  line L2500 (-87.5386, 199.641) -> (-91.8687, 197.141)
  line L2501 (-91.8687, 197.141) -> (-91.8687, 192.141)
  line L2502 (-91.8687, 192.141) -> (-87.5386, 189.641)
  line L2503 (-87.5386, 189.641) -> (-83.2084, 192.141)
  line L2504 (-83.2084, 192.141) -> (-83.2084, 197.141)
  line L2505 (-83.2084, 197.141) -> (-87.5386, 199.641)
  line L2506 (-76.8783, 199.641) -> (-81.2084, 197.141)
  line L2507 (-81.2084, 197.141) -> (-81.2084, 192.141)
  line L2508 (-81.2084, 192.141) -> (-76.8783, 189.641)
  line L2509 (-76.8783, 189.641) -> (-72.5482, 192.141)
  line L2510 (-72.5482, 192.141) -> (-72.5482, 197.141)
  line L2511 (-72.5482, 197.141) -> (-76.8783, 199.641)
  line L2512 (-66.218, 199.641) -> (-70.5482, 197.141)
  line L2513 (-70.5482, 197.141) -> (-70.5482, 192.141)
  line L2514 (-70.5482, 192.141) -> (-66.218, 189.641)
  line L2515 (-66.218, 189.641) -> (-61.8879, 192.141)
  line L2516 (-61.8879, 192.141) -> (-61.8879, 197.141)
  line L2517 (-61.8879, 197.141) -> (-66.218, 199.641)
  line L2518 (-55.5578, 199.641) -> (-59.8879, 197.141)
  line L2519 (-59.8879, 197.141) -> (-59.8879, 192.141)
  line L2520 (-59.8879, 192.141) -> (-55.5578, 189.641)
  line L2521 (-55.5578, 189.641) -> (-51.2277, 192.141)
  line L2522 (-51.2277, 192.141) -> (-51.2277, 197.141)
  line L2523 (-51.2277, 197.141) -> (-55.5578, 199.641)
  line L2524 (-44.8975, 199.641) -> (-49.2277, 197.141)
  line L2525 (-49.2277, 197.141) -> (-49.2277, 192.141)
  line L2526 (-49.2277, 192.141) -> (-44.8975, 189.641)
  line L2527 (-44.8975, 189.641) -> (-40.5674, 192.141)
  line L2528 (-40.5674, 192.141) -> (-40.5674, 197.141)
  line L2529 (-40.5674, 197.141) -> (-44.8975, 199.641)
  line L2530 (-34.2373, 199.641) -> (-38.5674, 197.141)
  line L2531 (-38.5674, 197.141) -> (-38.5674, 192.141)
  line L2532 (-38.5674, 192.141) -> (-34.2373, 189.641)
  line L2533 (-34.2373, 189.641) -> (-29.9072, 192.141)
  line L2534 (-29.9072, 192.141) -> (-29.9072, 197.141)
  line L2535 (-29.9072, 197.141) -> (-34.2373, 199.641)
  line L2536 (-23.577, 199.641) -> (-27.9072, 197.141)
  line L2537 (-27.9072, 197.141) -> (-27.9072, 192.141)
  line L2538 (-27.9072, 192.141) -> (-23.577, 189.641)
  line L2539 (-23.577, 189.641) -> (-19.2469, 192.141)
  line L2540 (-19.2469, 192.141) -> (-19.2469, 197.141)
  line L2541 (-19.2469, 197.141) -> (-23.577, 199.641)
  line L2542 (-12.9168, 199.641) -> (-17.2469, 197.141)
  line L2543 (-17.2469, 197.141) -> (-17.2469, 192.141)
  line L2544 (-17.2469, 192.141) -> (-12.9168, 189.641)
  line L2545 (-12.9168, 189.641) -> (-8.5866, 192.141)
  line L2546 (-8.5866, 192.141) -> (-8.5866, 197.141)
  line L2547 (-8.5866, 197.141) -> (-12.9168, 199.641)
  line L2548 (-2.2565, 199.641) -> (-6.5866, 197.141)
  line L2549 (-6.5866, 197.141) -> (-6.5866, 192.141)
  line L2550 (-6.5866, 192.141) -> (-2.2565, 189.641)
  line L2551 (-2.2565, 189.641) -> (2.0736, 192.141)
  line L2552 (2.0736, 192.141) -> (2.0736, 197.141)
  line L2553 (2.0736, 197.141) -> (-2.2565, 199.641)
  line L2554 (8.4037, 199.641) -> (4.0736, 197.141)
  line L2555 (4.0736, 197.141) -> (4.0736, 192.141)
  line L2556 (4.0736, 192.141) -> (8.4037, 189.641)
  line L2557 (8.4037, 189.641) -> (12.7339, 192.141)
  line L2558 (12.7339, 192.141) -> (12.7339, 197.141)
  line L2559 (12.7339, 197.141) -> (8.4037, 199.641)
  line L2560 (19.064, 199.641) -> (14.7339, 197.141)
  line L2561 (14.7339, 197.141) -> (14.7339, 192.141)
  line L2562 (14.7339, 192.141) -> (19.064, 189.641)
  line L2563 (19.064, 189.641) -> (23.3941, 192.141)
  line L2564 (23.3941, 192.141) -> (23.3941, 197.141)
  line L2565 (23.3941, 197.141) -> (19.064, 199.641)
  line L2566 (29.7242, 199.641) -> (25.3941, 197.141)
  line L2567 (25.3941, 197.141) -> (25.3941, 192.141)
  line L2568 (25.3941, 192.141) -> (29.7242, 189.641)
  line L2569 (29.7242, 189.641) -> (34.0544, 192.141)
  line L2570 (34.0544, 192.141) -> (34.0544, 197.141)
  line L2571 (34.0544, 197.141) -> (29.7242, 199.641)
  line L2572 (40.3845, 199.641) -> (36.0544, 197.141)
  line L2573 (36.0544, 197.141) -> (36.0544, 192.141)
  line L2574 (36.0544, 192.141) -> (40.3845, 189.641)
  line L2575 (40.3845, 189.641) -> (44.7146, 192.141)
  line L2576 (44.7146, 192.141) -> (44.7146, 197.141)
  line L2577 (44.7146, 197.141) -> (40.3845, 199.641)
  line L2578 (51.0447, 199.641) -> (46.7146, 197.141)
  line L2579 (46.7146, 197.141) -> (46.7146, 192.141)
  line L2580 (46.7146, 192.141) -> (51.0447, 189.641)
  line L2581 (51.0447, 189.641) -> (55.3749, 192.141)
  line L2582 (55.3749, 192.141) -> (55.3749, 197.141)
  line L2583 (55.3749, 197.141) -> (51.0447, 199.641)
  line L2584 (61.705, 199.641) -> (57.3749, 197.141)
  line L2585 (57.3749, 197.141) -> (57.3749, 192.141)
  line L2586 (57.3749, 192.141) -> (61.705, 189.641)
  line L2587 (61.705, 189.641) -> (66.0351, 192.141)
  line L2588 (66.0351, 192.141) -> (66.0351, 197.141)
  line L2589 (66.0351, 197.141) -> (61.705, 199.641)
  line L2590 (-146.17, 208.8731) -> (-150.5001, 206.3731)
  line L2591 (-150.5001, 206.3731) -> (-150.5001, 201.3731)
  line L2592 (-150.5001, 201.3731) -> (-146.17, 198.8731)
  line L2593 (-146.17, 198.8731) -> (-141.8398, 201.3731)
  line L2594 (-141.8398, 201.3731) -> (-141.8398, 206.3731)
  line L2595 (-141.8398, 206.3731) -> (-146.17, 208.8731)
  line L2596 (-135.5097, 208.8731) -> (-139.8398, 206.3731)
  line L2597 (-139.8398, 206.3731) -> (-139.8398, 201.3731)
  line L2598 (-139.8398, 201.3731) -> (-135.5097, 198.8731)
  line L2599 (-135.5097, 198.8731) -> (-131.1796, 201.3731)
  line L2600 (-131.1796, 201.3731) -> (-131.1796, 206.3731)
  line L2601 (-131.1796, 206.3731) -> (-135.5097, 208.8731)
  line L2602 (-124.8494, 208.8731) -> (-129.1796, 206.3731)
  line L2603 (-129.1796, 206.3731) -> (-129.1796, 201.3731)
  line L2604 (-129.1796, 201.3731) -> (-124.8494, 198.8731)
  line L2605 (-124.8494, 198.8731) -> (-120.5193, 201.3731)
  line L2606 (-120.5193, 201.3731) -> (-120.5193, 206.3731)
  line L2607 (-120.5193, 206.3731) -> (-124.8494, 208.8731)
  line L2608 (-114.1892, 208.8731) -> (-118.5193, 206.3731)
  line L2609 (-118.5193, 206.3731) -> (-118.5193, 201.3731)
  line L2610 (-118.5193, 201.3731) -> (-114.1892, 198.8731)
  line L2611 (-114.1892, 198.8731) -> (-109.8591, 201.3731)
  line L2612 (-109.8591, 201.3731) -> (-109.8591, 206.3731)
  line L2613 (-109.8591, 206.3731) -> (-114.1892, 208.8731)
  line L2614 (-103.5289, 208.8731) -> (-107.8591, 206.3731)
  line L2615 (-107.8591, 206.3731) -> (-107.8591, 201.3731)
  line L2616 (-107.8591, 201.3731) -> (-103.5289, 198.8731)
  line L2617 (-103.5289, 198.8731) -> (-99.1988, 201.3731)
  line L2618 (-99.1988, 201.3731) -> (-99.1988, 206.3731)
  line L2619 (-99.1988, 206.3731) -> (-103.5289, 208.8731)
  line L2620 (-92.8687, 208.8731) -> (-97.1988, 206.3731)
  line L2621 (-97.1988, 206.3731) -> (-97.1988, 201.3731)
  line L2622 (-97.1988, 201.3731) -> (-92.8687, 198.8731)
  line L2623 (-92.8687, 198.8731) -> (-88.5386, 201.3731)
  line L2624 (-88.5386, 201.3731) -> (-88.5386, 206.3731)
  line L2625 (-88.5386, 206.3731) -> (-92.8687, 208.8731)
  line L2626 (-82.2084, 208.8731) -> (-86.5386, 206.3731)
  line L2627 (-86.5386, 206.3731) -> (-86.5386, 201.3731)
  line L2628 (-86.5386, 201.3731) -> (-82.2084, 198.8731)
  line L2629 (-82.2084, 198.8731) -> (-77.8783, 201.3731)
  line L2630 (-77.8783, 201.3731) -> (-77.8783, 206.3731)
  line L2631 (-77.8783, 206.3731) -> (-82.2084, 208.8731)
  line L2632 (-71.5482, 208.8731) -> (-75.8783, 206.3731)
  line L2633 (-75.8783, 206.3731) -> (-75.8783, 201.3731)
  line L2634 (-75.8783, 201.3731) -> (-71.5482, 198.8731)
  line L2635 (-71.5482, 198.8731) -> (-67.218, 201.3731)
  line L2636 (-67.218, 201.3731) -> (-67.218, 206.3731)
  line L2637 (-67.218, 206.3731) -> (-71.5482, 208.8731)
  line L2638 (-60.8879, 208.8731) -> (-65.218, 206.3731)
  line L2639 (-65.218, 206.3731) -> (-65.218, 201.3731)
  line L2640 (-65.218, 201.3731) -> (-60.8879, 198.8731)
  line L2641 (-60.8879, 198.8731) -> (-56.5578, 201.3731)
  line L2642 (-56.5578, 201.3731) -> (-56.5578, 206.3731)
  line L2643 (-56.5578, 206.3731) -> (-60.8879, 208.8731)
  line L2644 (-50.2277, 208.8731) -> (-54.5578, 206.3731)
  line L2645 (-54.5578, 206.3731) -> (-54.5578, 201.3731)
  line L2646 (-54.5578, 201.3731) -> (-50.2277, 198.8731)
  line L2647 (-50.2277, 198.8731) -> (-45.8975, 201.3731)
  line L2648 (-45.8975, 201.3731) -> (-45.8975, 206.3731)
  line L2649 (-45.8975, 206.3731) -> (-50.2277, 208.8731)
  line L2650 (-39.5674, 208.8731) -> (-43.8975, 206.3731)
  line L2651 (-43.8975, 206.3731) -> (-43.8975, 201.3731)
  line L2652 (-43.8975, 201.3731) -> (-39.5674, 198.8731)
  line L2653 (-39.5674, 198.8731) -> (-35.2373, 201.3731)
  line L2654 (-35.2373, 201.3731) -> (-35.2373, 206.3731)
  line L2655 (-35.2373, 206.3731) -> (-39.5674, 208.8731)
  line L2656 (-28.9072, 208.8731) -> (-33.2373, 206.3731)
  line L2657 (-33.2373, 206.3731) -> (-33.2373, 201.3731)
  line L2658 (-33.2373, 201.3731) -> (-28.9072, 198.8731)
  line L2659 (-28.9072, 198.8731) -> (-24.577, 201.3731)
  line L2660 (-24.577, 201.3731) -> (-24.577, 206.3731)
  line L2661 (-24.577, 206.3731) -> (-28.9072, 208.8731)
  line L2662 (-18.2469, 208.8731) -> (-22.577, 206.3731)
  line L2663 (-22.577, 206.3731) -> (-22.577, 201.3731)
  line L2664 (-22.577, 201.3731) -> (-18.2469, 198.8731)
  line L2665 (-18.2469, 198.8731) -> (-13.9168, 201.3731)
  line L2666 (-13.9168, 201.3731) -> (-13.9168, 206.3731)
  line L2667 (-13.9168, 206.3731) -> (-18.2469, 208.8731)
  line L2668 (-7.5866, 208.8731) -> (-11.9168, 206.3731)
  line L2669 (-11.9168, 206.3731) -> (-11.9168, 201.3731)
  line L2670 (-11.9168, 201.3731) -> (-7.5866, 198.8731)
  line L2671 (-7.5866, 198.8731) -> (-3.2565, 201.3731)
  line L2672 (-3.2565, 201.3731) -> (-3.2565, 206.3731)
  line L2673 (-3.2565, 206.3731) -> (-7.5866, 208.8731)
  line L2674 (3.0736, 208.8731) -> (-1.2565, 206.3731)
  line L2675 (-1.2565, 206.3731) -> (-1.2565, 201.3731)
  line L2676 (-1.2565, 201.3731) -> (3.0736, 198.8731)
  line L2677 (3.0736, 198.8731) -> (7.4037, 201.3731)
  line L2678 (7.4037, 201.3731) -> (7.4037, 206.3731)
  line L2679 (7.4037, 206.3731) -> (3.0736, 208.8731)
  line L2680 (13.7339, 208.8731) -> (9.4037, 206.3731)
  line L2681 (9.4037, 206.3731) -> (9.4037, 201.3731)
  line L2682 (9.4037, 201.3731) -> (13.7339, 198.8731)
  line L2683 (13.7339, 198.8731) -> (18.064, 201.3731)
  line L2684 (18.064, 201.3731) -> (18.064, 206.3731)
  line L2685 (18.064, 206.3731) -> (13.7339, 208.8731)
  line L2686 (24.3941, 208.8731) -> (20.064, 206.3731)
  line L2687 (20.064, 206.3731) -> (20.064, 201.3731)
  line L2688 (20.064, 201.3731) -> (24.3941, 198.8731)
  line L2689 (24.3941, 198.8731) -> (28.7242, 201.3731)
  line L2690 (28.7242, 201.3731) -> (28.7242, 206.3731)
  line L2691 (28.7242, 206.3731) -> (24.3941, 208.8731)
  line L2692 (35.0544, 208.8731) -> (30.7242, 206.3731)
  line L2693 (30.7242, 206.3731) -> (30.7242, 201.3731)
  line L2694 (30.7242, 201.3731) -> (35.0544, 198.8731)
  line L2695 (35.0544, 198.8731) -> (39.3845, 201.3731)